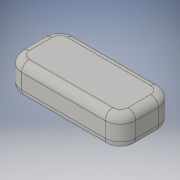
# Autodesk Inventor part: am-3277
Saved by Autodesk Inventor 2016 (Build 200138000, 138)
## iProperties
Created: 2015-10-22
Part Number: am-3277
Material: Generic
Document SubType Name: Modeling
Designer: TDM
Density: 2.36531 g/cm^3
Appearance: Default
Catalog Web Link: http://www.andymark.com/OM5P-AN-p/am-3277.htm
Description: Dual Band Radio, OM5P-AN Access Point
Vendor: AndyMark
Mass: 235.868 g
Surface Area: 132.938 cm^2
Volume: 99.7195 cm^3
Author: TDM
Autodesk Inventor part; units mm, degrees
ref_plane "YZ Plane" through (0, 0, 0) normal (1, 0, 0) x (0, 1, 0)
ref_plane "XZ Plane" through (0, 0, 0) normal (0, 1, 0) x (-1, 0, 0)
ref_plane "XY Plane" through (0, 0, 0) normal (0, 0, 1) x (1, 0, 0)
sketch "Sketch1" plane through (0, 0, 0) normal (0, 1, 0) x (-1, 0, 0)
  line L0 (-47.625, -22.225) -> (47.625, -22.225)
  line L1 (47.625, -22.225) -> (47.625, 22.225)
  line L2 (47.625, 22.225) -> (-47.625, 22.225)
  line L3 (-47.625, 22.225) -> (-47.625, -22.225)
  line L4 (-47.625, -22.225) -> (47.625, 22.225) construction
  line L5 (47.625, -22.225) -> (-47.625, 22.225) construction
  point P0 (0, 0)
  dimension "d0" = 95.25
  dimension "d1" = 44.45
  constraints: 12 end point, 2 midpoint, 2 parallel, 1 horizontal, 1 perpendicular
  measures "d0" distance of L2.end L1.end
  measures "d1" distance of L1.end L0.end
extrude "Extrusion1" add sketch "Sketch1" along normal blind 25.4
fillet "Fillet1" radius 12.7 4 edges at (-47.625, 12.7, 22.225) (47.625, 12.7, 22.225) (47.625, 12.7, -22.225) (-47.625, 12.7, -22.225)
fillet "Fillet2" radius 6.35 16 edges at (43.9053, 25.4, 18.5053) (47.625, 25.4, 0) (43.9053, 25.4, -18.5053) (0, 25.4, -22.225) (-43.9053, 25.4, -18.5053) (-47.625, 25.4, 0) (-43.9053, 25.4, 18.5053) (0, 25.4, 22.225) (43.9053, 0, 18.5053) (47.625, 0, 0) (43.9053, 0, -18.5053) (0, 0, -22.225) (-43.9053, 0, -18.5053) (-47.625, 0, 0) (-43.9053, 0, 18.5053) (0, 0, 22.225)
body "Solid1"
